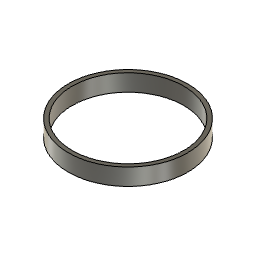
quarter 0.075 tolerance v1 (Autodesk Fusion 360 design; units mm, degrees)
Autodesk Fusion 360 part; units mm, degrees
sketch "Sketch1" plane through (0, 0, 0) normal (0, 0, 1) x (1, 0, 0)
  circle A0 centre (0, 0) radius 13.5255
  dimension "d1" = 27.051
  constraint coincident A0.centre origin
  measures "d1" diameter of A0
extrude "Extrude1" add sketch "Sketch1" along normal blind 3.81
shell "Shell1" thickness 0.889 removed faces 2 at (5.2851, -4.4959, 3.81) at (5.2851, -4.4959, 0)
